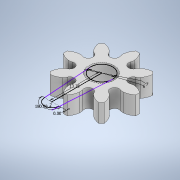
# Autodesk Inventor part: joint1
Saved by Autodesk Inventor 2020.2 (Build 242310000, 310)
## iProperties
Created: 2026-05-18
Part Number: joint1
Material: Generic
Document SubType Name: Modeling
Designer: explorer
Density: 1 g/cm^3
Appearance: Default
Author: explorer
Autodesk Inventor part; units mm, degrees
ref_plane "YZ Plane" through (0, 0, 0) normal (1, 0, 0) x (0, 1, 0)
ref_plane "XZ Plane" through (0, 0, 0) normal (0, 1, 0) x (-1, 0, 0)
ref_plane "XY Plane" through (0, 0, 0) normal (0, 0, 1) x (1, 0, 0)
sketch "Sketch7" plane through (0, 0, 0) normal (0, 1, 0) x (-1, 0, 0)
  circle A0 centre (0, 0) radius 3.5
  circle A1 centre (0, 0) radius 6.7
  circle A2 centre (6.7, 0) radius 1.25
  line L0 (0, 0) -> (5.4447, 5.4447)
  line L1 (0, 0) -> (7.7, 0) construction
  circle A3 centre (5.4447, 5.4447) radius 4.5
  dimension "d17" = 7
  dimension "d18" = 2.5
  dimension "d20" = 6.7
  dimension "d21" = 7.7
  dimension "d22" = 45
  dimension "d23" = 9
  constraints: 4 end point, 3 centre point, 3 coincident, 1 equal length, 1 horizontal, 1 horizontal alignment, 2 other
  measures "d17" diameter of A0
  measures "d18" diameter of A2
  measures "d20" distance of point (0, 0) A2.centre
  measures "d21" distance of L0.start L0.end
  measures "d22" angle of L1 L0
  measures "d23" diameter of A3
sketch "Sketch9" plane through (0, 0, 0) normal (0, 1, 0) x (-1, 0, 0)
  circle A0 centre (0, 0) radius 3.5
  circle A1 centre (0, 0) radius 6.7
  line L0 (0, 0) -> (7.1139, -2.9467)
  line L1 (0, 0) -> (2.9467, -7.1139) construction
  circle A2 centre (7.1139, -2.9467) radius 4.5
  circle A3 centre (0, 0) radius 10
  circle A4 centre (6.19, -2.564) radius 1.25
  circle A5 centre (7.1139, 2.9467) radius 4.5
  circle A6 centre (6.19, 2.564) radius 1.25
  circle A7 centre (2.9467, 7.1139) radius 4.5
  circle A8 centre (2.564, 6.19) radius 1.25
  circle A9 centre (-2.9467, 7.1139) radius 4.5
  circle A10 centre (-2.564, 6.19) radius 1.25
  circle A11 centre (-7.1139, 2.9467) radius 4.5
  circle A12 centre (-6.19, 2.564) radius 1.25
  circle A13 centre (-7.1139, -2.9467) radius 4.5
  circle A14 centre (-6.19, -2.564) radius 1.25
  circle A15 centre (-2.9467, -7.1139) radius 4.5
  circle A16 centre (-2.564, -6.19) radius 1.25
  circle A17 centre (2.9467, -7.1139) radius 4.5
  line L2 (-7.4352, -7.4352) -> (0, 0)
  circle A18 centre (2.564, -6.19) radius 1.25
  point P0 (5.0895, 3.1568)
  point P1 (7.4272, 6.696)
  point P2 (9.9866, -0.517)
  point P3 (3.1568, 5.0895)
  point P4 (1.3666, 5.8311)
  point P5 (0.517, 9.9866)
  point P6 (-0.517, 9.9866)
  point P7 (-1.3666, 5.8311)
  point P8 (-3.1568, 5.0895)
  point P9 (-6.696, 7.4272)
  point P10 (-7.4272, 6.696)
  point P11 (-5.0895, 3.1568)
  point P12 (-5.8311, 1.3666)
  point P13 (-9.9866, 0.517)
  point P14 (-9.9866, -0.517)
  point P15 (-5.8311, -1.3666)
  point P16 (-5.0895, -3.1568)
  point P17 (-7.4272, -6.696)
  point P18 (-6.696, -7.4272)
  point P19 (-3.7976, -5.9885)
  point P20 (-1.3666, -5.8311)
  point P21 (7.4272, -6.696)
  point P22 (0.517, -9.9866)
  point P23 (6.696, -7.4272)
  point P24 (-0.517, -9.9866)
  point P25 (5.9885, -3.7976)
  point P26 (5.8311, -1.3666)
  point P27 (6.696, 7.4272)
  point P28 (9.9866, 0.517)
  point P29 (5.8311, 1.3666)
  point P30 (7.4352, -7.4352)
  point P31 (10.5149, 0)
  point P32 (0, -10.5149)
  point P33 (3.7128, 0)
  point P34 (3.4887, -0.2805)
  point P35 (2.6653, -2.2686)
  point P36 (2.6254, -2.6254)
  point P37 (2.2686, -2.6653)
  point P38 (0.2805, -3.4887)
  point P39 (0, -3.7128)
  point P40 (-0.2805, -3.4887)
  point P41 (-2.2686, -2.6653)
  point P42 (-2.6254, -2.6254)
  point P43 (-2.6653, -2.2686)
  point P44 (-3.4887, -0.2805)
  point P45 (-3.7128, 0)
  point P46 (-3.4887, 0.2805)
  point P47 (-2.6653, 2.2686)
  point P48 (-2.6254, 2.6254)
  point P49 (-2.2686, 2.6653)
  point P50 (-0.2805, 3.4887)
  point P51 (0, 3.7128)
  point P52 (0.2805, 3.4887)
  point P53 (2.2686, 2.6653)
  point P54 (2.6254, 2.6254)
  point P55 (2.6653, 2.2686)
  point P56 (3.4887, 0.2805)
  point P57 (3.7976, -5.9885)
  point P58 (6.9198, -1.5492)
  point P59 (6.9198, 1.5492)
  point P60 (5.9885, 3.7976)
  point P61 (3.7976, 5.9885)
  point P62 (1.5492, 6.9198)
  point P63 (-1.5492, 6.9198)
  point P64 (-3.7976, 5.9885)
  point P65 (-5.9885, 3.7976)
  point P66 (-6.9198, 1.5492)
  point P67 (-6.9198, -1.5492)
  point P68 (-5.9885, -3.7976)
  point P69 (-1.5492, -6.9198)
  point P70 (1.5492, -6.9198)
  dimension "d36" = 360
  dimension "d43" = 45
  constraints: 17 centre point, 6 end point, 4 coincident, 1 equal length, 10 other
extrude "Extrusion2" add sketch "Sketch9" along normal blind 5 contours A0 A5 A2 | A0 A5 A7 A6 A2 | A2 A5 A4 L0 A0 | A0 A7 A5 | A2 A6 A1 A4 A5 | L0 A4 A17 A2 A0 | A0 A7 A9 A8 A5 | A5 A8 A1 A6 A7 | A2 A17 A0 | A0 A9 A7 | A6 A2 A3 A5 A4 A1 | A17 A2 A18 A15 A0 | A17 A4 A1 A18 A2 | L2 A13 A0 | A0 A15 L2 | A0 A9 A11 A10 A7 | A7 A10 A1 A8 A9 | A8 A5 A3 A7 A6 A1 | A17 A15 A0 | A4 A17 A3 A2 A18 A1 | A13 A15 A14 A11 A0 | A0 A15 A17 A16 A13 | L2 A1 A14 A15 | A13 A16 A1 L2 | A0 A11 A9 | A1 A10 A7 A3 A9 A8 | A15 A18 A1 A16 A17 | A13 A11 A0 | L2 A3 A15 A14 A1 | A1 A16 A13 A3 L2 | A0 A11 A13 A12 A9 | A9 A12 A1 A10 A11 | A18 A15 A3 A17 A16 A1 | A11 A14 A1 A12 A13 | A1 A12 A9 A3 A11 A10 | A14 A11 A3 A13 A12 A1
fillet "Fillet3" radius 2 16 edges at (-5.9885, 2.5, 3.7976) (-6.9198, 2.5, 1.5492) (-6.9198, 2.5, -1.5492) (-5.9885, 2.5, -3.7976) (-3.7976, 2.5, -5.9885) (-1.5492, 2.5, -6.9198) (1.5492, 2.5, -6.9198) (3.7976, 2.5, -5.9885) (5.9885, 2.5, -3.7976) (6.9198, 2.5, -1.5492) (6.9198, 2.5, 1.5492) (5.9885, 2.5, 3.7976) (3.7976, 2.5, 5.9885) (1.5492, 2.5, 6.9198) (-1.5492, 2.5, 6.9198) (-3.7976, 2.5, 5.9885)
sketch "Sketch10" plane through (0, 5, 0) normal (0, 1, 0) x (1, 0, 0)
  circle A0 centre (0, 0) radius 3.5 construction
  circle A1 centre (0, 0) radius 3
  line L0 (0, 0) -> (0, -13.75)
  arc A2 (-2, -13.75) -> (2, -13.75) centre (0, -13.75) ccw
  line L1 (0, -13.75) -> (2, -13.75) construction
  line L2 (0, -13.75) -> (2, -13.75) construction
  line L3 (0, -13.75) -> (-2, -13.75) construction
  line L4 (3, 0) -> (2, -15.75)
  line L5 (-3, 0) -> (-2, -13.75)
  dimension "d46" = 7
  dimension "d47" = 6
  dimension "d48" = 13.75
  dimension "d49" = 2
  dimension "d50" = 0
  dimension "d51" = 180
  constraints: 12 end point, 4 point on circle, 3 centre point, 3 coincident, 1 collinear, 1 horizontal, 1 vertical
  measures "d46" diameter of A0
  measures "d47" diameter of A1
  measures "d48" distance of L0.start L0.end
  measures "d49" radius of A2
  measures "d50" distance between parallel lines of L1 L2
  measures "d51" angle of L1 L3
body "Solid2"
